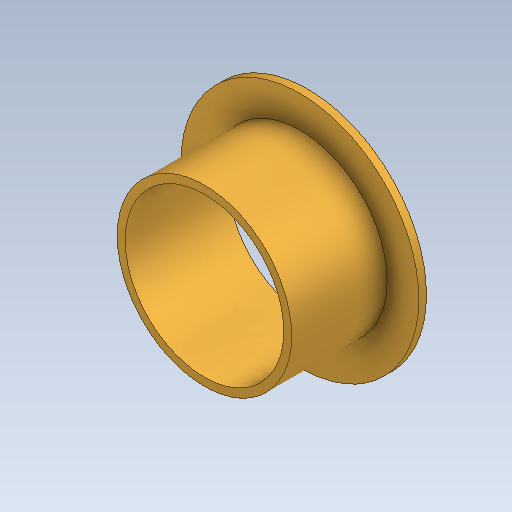
# Autodesk Inventor part: ドライメッシュw6.5f10-11a
Saved by Autodesk Inventor 2020 (Build 240168000, 168)
## iProperties
Created: 2020-04-10
Part Number: ドライメッシュw6.5f10-11a
Material: 真鍮、ソフト イエロー
Document SubType Name: Modeling
Designer: happy
Density: 8.47 g/cm^3
Appearance: 真鍮 - サテン
Mass: 1.24013 g
Surface Area: 6.31209 cm^2
Volume: 0.146414 cm^3
Author: happy
Autodesk Inventor part; units mm, degrees
ref_plane "YZ Plane" through (0, 0, 0) normal (1, 0, 0) x (0, 1, 0)
ref_plane "XZ Plane" through (0, 0, 0) normal (0, 1, 0) x (-1, 0, 0)
ref_plane "XY Plane" through (0, 0, 0) normal (0, 0, 1) x (1, 0, 0)
sketch "スケッチ1" plane through (0, 0, 0) normal (0, 0, 1) x (1, 0, 0)
  circle A0 centre (0, 0) radius 5
  circle A1 centre (0, 0) radius 5.5
  circle A2 centre (0, 0) radius 7.5
  dimension "d0" = 10
  dimension "d1" = 11
  dimension "d4" = 15
  constraints: 3 centre point, 3 coincident
  measures "d0" diameter of A0
  measures "d1" diameter of A1
  measures "d4" diameter of A2
extrude "押し出し1" add sketch "スケッチ1" along normal blind 6.5 contours A1
extrude "押し出し2" add sketch "スケッチ1" along normal blind 0.48 contours A2
